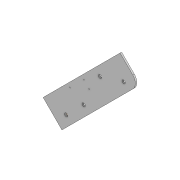
# Autodesk Inventor part: new sidewall outside
Saved by Autodesk Inventor 2020 (Build 240168000, 168)
## iProperties
Created: 2020-02-26
Part Number: new sidewall outside
Material: Generic
Document SubType Name: Modeling
Designer: jackm
Density: 1 g/cm^3
Appearance: Default
Author: jackm
Autodesk Inventor part; units mm, degrees
ref_plane "YZ Plane" through (0, 0, 0) normal (1, 0, 0) x (0, 1, 0)
ref_plane "XZ Plane" through (0, 0, 0) normal (0, 1, 0) x (-1, 0, 0)
ref_plane "XY Plane" through (0, 0, 0) normal (0, 0, 1) x (1, 0, 0)
ref_plane "Work Plane1" through (-237.6364, -237.6364, 0) normal (0, 0, 1) x (0.7071, 0.7071, 0)
sketch "Sketch1" plane through (-237.6364, -237.6364, 0) normal (0, 0, 1) x (0.7071, 0.7071, 0)
  circle A0 centre (0, 0) radius 4.15 construction
  circle A1 centre (336.0686, 0) radius 6.45 construction
  circle A2 centre (246.0297, 47.9271) radius 4.83 construction
  circle A3 centre (102, -0.0729) radius 4.83 construction
  circle A4 centre (0, 0) radius 6.8857
  circle A5 centre (336.0686, 0) radius 6.8834
  circle A6 centre (102, -0.0729) radius 6.8834
  circle A7 centre (246.0297, 47.9271) radius 6.8834
  line L0 (78.0149, 71.9271) -> (270.0149, 71.9271) construction
  line L1 (168.0343, 78.2771) -> (168.0343, 71.9271)
  line L2 (168.0343, 78.2771) -> (393.4593, 78.2771)
  line L3 (168.0343, 78.2771) -> (-57.3907, 78.2771)
  line L4 (-57.3907, -31.75) -> (-57.3907, 78.2771)
  line L5 (-57.3907, -31.75) -> (358.1679, -31.75)
  line L6 (393.4593, 3.5414) -> (393.4593, 78.2771)
  arc A8 (358.1679, -31.75) -> (393.4593, 3.5414) centre (358.1679, 3.5414) ccw
  point P0 (336.0686, 0)
  dimension "d0" = 13.7714
  dimension "d1" = 13.7668
  dimension "d2" = 13.7668
  dimension "d3" = 13.7668
  dimension "d6" = 225.425
  dimension "d7" = 225.425
  constraints: 12 end point, 5 centre point, 4 coincident, 3 horizontal, 2 perpendicular, 2 point on circle, 1 point on line
  measures "d0" diameter of A4
  measures "d1" diameter of A5
  measures "d2" diameter of A6
  measures "d3" diameter of A7
  measures "d6" distance of L1.start L2.end
  measures "d7" distance of L1.start L3.end
extrude "Extrusion1" add sketch "Sketch1" along normal blind 6.35
sketch "Sketch3" plane through (-237.6364, -237.6364, 6.35) normal (0, 0, 1) x (0.7071, -0.7071, 0)
  circle A0 centre (-63.9271, 166.0149) radius 3.81 construction
  circle A1 centre (-31.9271, 166.0149) radius 3.81 construction
  circle A2 centre (-15.9271, 166.0149) radius 3.81 construction
  circle A3 centre (-63.9271, 86.0149) radius 3.81 construction
  circle A4 centre (16.0729, 166.0149) radius 3.81 construction
  circle A5 centre (-31.9271, 166.0149) radius 3.81 construction
  circle A6 centre (-63.9271, 86.0149) radius 5.08 construction
  circle A7 centre (-31.9271, 86.0149) radius 3.81 construction
  circle A8 centre (-15.9271, 86.0149) radius 3.81 construction
  circle A9 centre (16.0729, 86.0149) radius 3.81 construction
  circle A10 centre (-63.9271, 86.0149) radius 1.778
  circle A11 centre (-31.9271, 166.0149) radius 1.778
  circle A12 centre (-63.9271, 166.0149) radius 1.778
  circle A13 centre (16.0729, 166.0149) radius 1.9304 construction
  circle A14 centre (16.0729, 246.0149) radius 1.9304 construction
  circle A15 centre (-15.9271, 166.0149) radius 1.9304 construction
  circle A16 centre (16.0729, 246.0149) radius 1.778
  point P0 (0, 336.0686)
  dimension "d11" = 3.556
  dimension "d17" = 3.556
  dimension "d18" = 3.556
  dimension "d21" = 3.556
  constraints: 4 centre point, 4 coincident
  measures "d11" diameter of A10
  measures "d17" diameter of A11
  measures "d18" diameter of A12
  measures "d21" diameter of A16
extrude "Extrusion2" cut sketch "Sketch3" against normal through all contours A10 | A11 | A12
body "Solid1"
